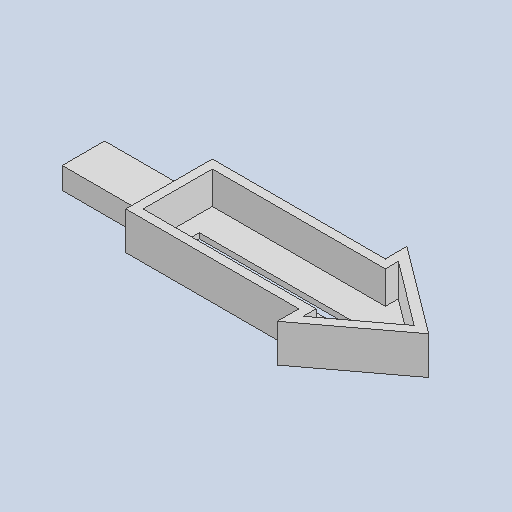
# Autodesk Inventor part: Part_5_ledholder
Saved by Autodesk Inventor 2023 (Build 270158000, 158)
## iProperties
Created: 2023-10-01
Part Number: Part_5_ledholder
Material: Generic
Document SubType Name: Modeling
Designer: zskus
Density: 1 g/cm^3
Appearance: Default
Author: zskus
Autodesk Inventor part; units mm, degrees
ref_plane "YZ Plane" through (0, 0, 0) normal (1, 0, 0) x (0, 1, 0)
ref_plane "XZ Plane" through (0, 0, 0) normal (0, 1, 0) x (-1, 0, 0)
ref_plane "XY Plane" through (0, 0, 0) normal (0, 0, 1) x (1, 0, 0)
sketch "Sketch1" plane through (0, 0, 0) normal (0, 1, 0) x (-1, 0, 0)
  line L0 (12.573, 6.223) -> (-12.573, 6.223)
  line L1 (-12.573, 6.223) -> (-12.573, -6.223)
  line L2 (-12.573, -6.223) -> (12.573, -6.223)
  line L3 (12.573, -6.223) -> (12.573, 6.223)
  point P0 (0, 0)
  dimension "d0" = 12.446
  dimension "d1" = 25.146
  dimension "d2" = 6.223
  dimension "d3" = 12.573
  constraints: 8 end point, 2 parallel, 1 horizontal, 1 perpendicular
  measures "d0" distance of L2.end L0.start
  measures "d1" distance of L1.end L2.end
  measures "d2" distance from line of L2 point (0, 0)
  measures "d3" distance from line of point (0, 0) L3
extrude "Extrusion1" add sketch "Sketch1" along normal blind 6.35
sketch "Sketch2" plane through (12.573, 0, 6.223) normal (1, 0, 0) x (0, 0, -1)
  line L0 (-6.477, 0) -> (18.923, 0)
  line L1 (18.923, 0) -> (18.923, 1.5875)
  line L2 (18.923, 1.5875) -> (-6.477, 1.5875)
  line L3 (-6.477, 1.5875) -> (-6.477, 0)
  line L4 (0, 0) -> (12.446, 0) projected
  line L5 (0, 0) -> (12.446, 0) projected
  line L6 (12.446, 0) -> (12.446, 6.35) projected
  line L7 (0, 6.35) -> (12.446, 6.35) projected
  line L8 (0, 0) -> (0, 6.35) projected
  point P0 (6.223, 0)
  point P1 (6.223, 0)
  dimension "d6" = 25.4
  dimension "d7" = 12.7
  dimension "d8" = 1.5875
  constraints: 8 end point, 2 parallel, 1 horizontal, 1 midpoint, 1 perpendicular, 1 point on line
  measures "d6" distance of L1.end L2.end
  measures "d7" horizontal distance of point (6.223, 0) L1.end
  measures "d8" distance of L0.end L1.end
extrude "Extrusion2" add sketch "Sketch2" along normal blind 50.8 contours L3 L2 L8 L0 | L8 L2 L6 L0 | L6 L2 L1 L0
sketch "Sketch3" plane through (12.573, 1.5875, -6.223) normal (0, 1, 0) x (1, 0, 0)
  line L0 (0, 6.477) -> (0, 0) projected
  line L1 (0, -12.446) -> (0, 0) projected
  line L2 (0, -12.446) -> (0, -18.923) projected
  line L3 (0, -18.923) -> (50.8, -18.923) projected
  line L4 (50.8, 6.477) -> (50.8, -18.923) projected
  line L5 (0, 6.477) -> (50.8, 6.477) projected
  line L6 (50.8, -25.273) -> (50.8, 12.827)
  line L7 (50.8, 12.827) -> (76.2, -6.223)
  line L8 (76.2, -6.223) -> (50.8, -25.273)
  point P0 (-12.573, -6.223)
  point P1 (50.8, -18.923)
  dimension "d11" = 38.1
  dimension "d12" = 6.35
  dimension "d13" = 12.7
  dimension "d14" = 12.7
  dimension "d15" = 25.4
  dimension "d16" = 50.8
  dimension "d17" = 50.8
  constraints: 6 end point
  measures "d11" distance of L6.start L6.end
  measures "d12" distance from line of L3 L6.start
  measures "d13" distance from line of L5 L7.end
  measures "d14" distance from line of L3 L7.end
  measures "d15" distance from line of L4 L7.end
  measures "d16" distance of L2.end L3.end
  measures "d17" distance between parallel lines of L1 L6
extrude "Extrusion3" add sketch "Sketch3" against normal blind 1.5875 contours L6 L7 L8 L4
sketch "Sketch4" plane through (12.573, 1.5875, -6.223) normal (0, 1, 0) x (1, 0, 0)
  line L0 (0, 6.477) -> (0, 0) projected
  line L1 (0, -12.446) -> (0, 0) projected
  line L2 (0, -12.446) -> (0, -18.923) projected
  line L3 (0, -18.923) -> (50.8, -18.923) projected
  line L4 (50.8, -18.923) -> (50.8, -25.273) projected
  line L5 (50.8, -25.273) -> (76.2, -6.223) projected
  line L6 (76.2, -6.223) -> (50.8, 12.827) projected
  line L7 (50.8, 12.827) -> (50.8, 6.477) projected
  line L8 (0, 6.477) -> (50.8, 6.477) projected
  line L9 (53.34, 3.937) -> (53.34, 7.747)
  line L10 (53.34, 7.747) -> (71.9667, -6.223)
  line L11 (71.9667, -6.223) -> (53.34, -20.193)
  line L12 (53.34, -20.193) -> (53.34, -16.383)
  line L13 (53.34, -16.383) -> (2.54, -16.383)
  line L14 (2.54, -16.383) -> (2.54, -12.446)
  line L15 (2.54, -12.446) -> (2.54, 0)
  line L16 (2.54, 0) -> (2.54, 3.937)
  line L17 (2.54, 3.937) -> (53.34, 3.937)
  point P0 (-12.573, -6.223)
  dimension "d20" = 2.54
  constraints: 18 end point, 8 other
  measures "d20" distance between parallel lines of L8 L17
extrude "Extrusion4" add sketch "Sketch4" along normal blind 9.525
sketch "Sketch6" plane through (15.113, 1.5875, -10.16) normal (0, 1, 0) x (1, 0, 0)
  line L0 (4.7625, -8.5725) -> (58.7375, -8.5725)
  line L1 (58.7375, -8.5725) -> (58.7375, -11.7475)
  line L2 (58.7375, -11.7475) -> (4.7625, -11.7475)
  line L3 (4.7625, -11.7475) -> (4.7625, -8.5725)
  line L4 (-27.686, -3.937) -> (-27.686, -16.383) projected
  point P0 (-15.113, -10.16)
  point P1 (-27.686, -10.16)
  dimension "d23" = 3.175
  dimension "d24" = 1.5875
  constraints: 8 end point, 2 parallel, 1 horizontal, 1 midpoint, 1 perpendicular
  measures "d23" distance between parallel lines of L2 L0
  measures "d24" distance from line of point (-27.686, -10.16) L0
extrude "Extrusion5" cut sketch "Sketch6" against normal blind 9.525
equation "\"d2\" = 0.5 * d0"
equation "\"d3\" = 0.5 * d1"
equation "\"d7\" = 0.5 * d6"
equation "\"d17\" = d16"
equation "\"d24\" = 0.5 * d23"
body "Solid1"
